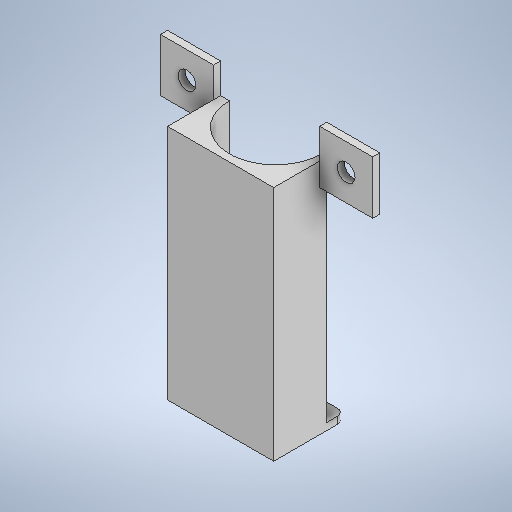
# Autodesk Inventor part: Motorhalterung
Saved by Autodesk Inventor 2025.1 (Build 291241000, 241)
## iProperties
Created: 2024-12-18
Part Number: Motorhalterung
Material: Generisch
Document SubType Name: Modeling
Designer: Julian
Density: 1 g/cm^3
Appearance: Vorgabe
Author: Julian
Autodesk Inventor part; units mm, degrees
ref_plane "YZ Plane" through (0, 0, 0) normal (1, 0, 0) x (0, 1, 0)
ref_plane "XZ Plane" through (0, 0, 0) normal (0, 1, 0) x (-1, 0, 0)
ref_plane "XY Plane" through (0, 0, 0) normal (0, 0, 1) x (1, 0, 0)
sketch "Skizze1" plane through (0, 0, 0) normal (0, 0, 1) x (1, 0, 0)
  line L0 (15, 7.5) -> (15, -7.5)
  line L1 (15, -7.5) -> (-15, -7.5)
  line L2 (-15, -7.5) -> (-15, 7.5)
  line L3 (-15, 7.5) -> (15, -7.5) construction
  line L4 (15, 7.5) -> (-15, -7.5) construction
  arc A0 (-12.5, 7.5) -> (13.5, 7.5) centre (0.5, 7.5) ccw
  line L5 (-15, 7.5) -> (-12.5, 7.5)
  line L6 (13.5, 7.5) -> (15, 7.5)
  point P0 (0, 0)
  dimension "d0" = 30
  dimension "d1" = 15
  dimension "d2" = 26
  constraints: 14 end point, 3 parallel, 2 horizontal, 2 midpoint, 2 perpendicular, 2 point on circle, 1 centre point
  measures "d0" distance of L0.end L1.end
  measures "d1" distance of L0.start L0.end
  measures "d2" diameter of A0
extrude "Extrusion1" add sketch "Skizze1" along normal blind 65
sketch "Skizze2" plane through (0, 0, 65) normal (0, 0, 1) x (1, 0, 0)
  line L0 (-15, 7.5) -> (-15, -7.5) projected
  line L1 (15, 7.5) -> (13.5, 7.5) projected
  line L2 (-15, -7.5) -> (15, -7.5)
  line L3 (15, -7.5) -> (15, 7.5)
  line L4 (-15, 7.5) -> (-15, -7.5)
  arc A0 (-12.5, 7.5) -> (13.5, 7.5) centre (0.5, 7.5) ccw projected
  arc A1 (0, -5.4904) -> (13.5, 7.5) centre (0.5, 7.5) ccw
  arc A2 (-12.5, 7.5) -> (0, -5.4904) centre (0.5, 7.5) ccw
  point P0 (0, 0)
  constraints: 6 end point, 5 point on circle, 2 centre point, 1 concentric, 1 horizontal, 1 parallel, 1 perpendicular
extrude "Extrusion2" [suppressed]
sketch "Skizze3" plane through (0, 0, 67) normal (0, 0, 1) x (1, 0, 0)
  line L0 (-15, 7.5) -> (-15, -7.5) projected
  line L1 (-15, -7.5) -> (15.179, -7.5)
  line L2 (15.179, -7.5) -> (15.179, 7.5)
  line L3 (15.179, 7.5) -> (-15, 7.5)
  line L4 (-15, 7.5) -> (-15, -7.5)
  arc A0 (-12.9105, 7.5) -> (13.0895, 7.5) centre (0.0895, 7.5) ccw
  point P0 (0, 0)
  dimension "d7" = 26
  constraints: 8 end point, 2 parallel, 2 point on circle, 2 point on line, 1 centre point, 1 horizontal, 1 midpoint, 1 perpendicular
  measures "d7" diameter of A0
extrude "Extrusion3" [suppressed]
sketch "Skizze4" plane through (0, 0, 132) normal (0, 0, 1) x (1, 0, 0)
  line L0 (-15, 7.5) -> (-15, -7.5) projected
  line L1 (-15, -7.5) -> (15, -7.5)
  line L2 (15, -7.5) -> (15, 12.5)
  line L3 (15, 12.5) -> (-15, 12.5)
  line L4 (-15, 12.5) -> (-15, -7.5)
  point P0 (0, 0)
  dimension "d10" = 30
  dimension "d11" = 20
  constraints: 8 end point, 2 parallel, 1 horizontal, 1 perpendicular
  measures "d10" distance of L3.end L2.end
  measures "d11" distance of L2.end L1.end
extrude "Extrusion4" [suppressed]
sketch "Skizze5" plane through (0, 0, 134) normal (0, 0, 1) x (1, 0, 0)
  circle A0 centre (0, 7.5) radius 2.5
  point P0 (0, 0)
  dimension "d14" = 5
  constraints: 1 centre point
  measures "d14" diameter of A0
extrude "Extrusion5" [suppressed]
sketch "Skizze6" plane through (0, 0, 0) normal (0, 0, -1) x (-1, 0, 0)
  line L0 (-15.179, -7.5) -> (-15, -7.5) projected
  line L1 (-15, 12.5) -> (15, 12.5) projected
  line L2 (-15, -7.5) -> (15, -7.5)
  line L3 (15, -7.5) -> (15, 12.5)
  line L4 (15, 12.5) -> (-15, 12.5)
  line L5 (-15, 12.5) -> (-15, -7.5)
  point P0 (0, 0)
  point P1 (-14.9426, -7.5)
  constraints: 8 end point, 2 parallel, 1 horizontal, 1 perpendicular
extrude "Extrusion6" add sketch "Skizze6" along normal blind 2
sketch "Skizze7" plane through (0, 0, -2) normal (0, 0, -1) x (-1, 0, 0)
  line L0 (-13.0895, 7.5) -> (12.9105, 7.5) projected
  circle A0 centre (0, 7.5) radius 2.5
  point P0 (0, 0)
  dimension "d19" = 5
  constraints: 1 centre point, 1 point on line
  measures "d19" diameter of A0
extrude "Extrusion7" cut sketch "Skizze7" against normal blind 2
fillet "Rundung1" radius 2 1 edges at (-15, 12.5, -1)
fillet "Rundung2" [suppressed]
fillet "Rundung3" [suppressed]
fillet "Rundung4" radius 2 1 edges at (15, 12.5, -1)
sketch "Skizze8" plane through (-15, -7.5, -2) normal (-1, 0, 0) x (0, 0, 1)
  line L0 (69, 0) -> (69, 15) projected
  line L1 (69, 15) -> (68, 15)
  line L2 (75.5, 13) -> (60.5, 13)
  line L3 (60.5, 13) -> (60.5, 15)
  line L4 (75.5, 15) -> (75.5, 13)
  line L5 (75.5, 13) -> (60.5, 17) construction
  line L6 (60.5, 13) -> (68, 15) construction
  line L7 (2, 15) -> (67, 15) projected
  line L8 (60.5, 15) -> (75.5, 15)
  point P0 (2, 7.5)
  dimension "d26" = 1
  dimension "d28" = 4
  constraints: 14 end point, 2 horizontal, 1 midpoint, 1 parallel, 1 perpendicular, 1 point on line
  measures "d26" distance of L1.end L0.end
  measures "d28" distance of L2.end L5.end
extrude "Extrusion8" add sketch "Skizze8" along normal blind 15
sketch "Skizze9" plane through (-12.5, 7.5, 65) normal (0, 1, 0) x (1, 0, 0)
  line L0 (-2.5, 6.5) -> (-17.5, 6.5) projected
  line L1 (-2.5, 67) -> (-2.5, 0) projected
  line L2 (-17.5, 6.5) -> (3.7132, 6.5) construction
  circle A0 centre (-10, -1) radius 2.5
  point P0 (12.5, 65)
  point P1 (-2.5, -69)
  dimension "d32" = 5
  constraints: 2 end point, 1 centre point, 1 horizontal
  measures "d32" diameter of A0
extrude "Extrusion9" cut sketch "Skizze9" against normal through all
sketch "Skizze10" plane through (15, -7.5, 67) normal (1, 0, 0) x (0, 0, -1)
  line L0 (0, 15) -> (1, 15)
  line L1 (67, 15) -> (2, 15) projected
  line L2 (8.5, 17) -> (-6.5, 17)
  line L3 (-6.5, 15) -> (-6.5, 13)
  line L4 (-6.5, 13) -> (8.5, 13)
  line L5 (8.5, 13) -> (8.5, 15)
  line L6 (1, 15) -> (-6.5, 13) construction
  line L7 (1, 15) -> (8.5, 13) construction
  line L8 (0, 15) -> (-65, 15) projected
  line L9 (-6.5, 15) -> (8.5, 15)
  point P0 (67, 7.5)
  point P1 (8.5, 15)
  point P2 (1, 15)
  dimension "d35" = 1
  dimension "d37" = 4
  constraints: 16 end point, 2 parallel, 2 point on line, 1 horizontal, 1 perpendicular
  measures "d35" distance of L0.end L0.start
  measures "d37" distance of L3.end L2.end
extrude "Extrusion10" add sketch "Skizze10" along normal blind 15
sketch "Skizze11" plane through (-12.5, 7.5, 65) normal (0, 1, 0) x (1, 0, 0)
  line L0 (27.679, -8.5) -> (27.679, -67) projected
  line L1 (42.5, -8.5) -> (42.5, 6.5) projected
  line L2 (27.679, -8.5) -> (48.6391, -8.5) construction
  line L3 (27.5, 6.5) -> (27.5, 0) projected
  circle A0 centre (35, -1) radius 2.5
  point P0 (12.5, 65)
  point P1 (27.5, -2)
  dimension "d41" = 5
  constraints: 2 end point, 1 centre point, 1 horizontal
  measures "d41" diameter of A0
extrude "Extrusion11" cut sketch "Skizze11" against normal through all
